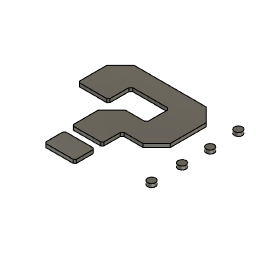
Question (Autodesk Fusion 360 design; units mm, degrees)
Autodesk Fusion 360 part; units mm, degrees
(part 1 of 2)
sketch "Schizzo1" plane through (0, 0, 0) normal (0, 0, 1) x (1, 0, 0)
  line L0 (0, 0) -> (90, 0)
  line L1 (90, 0) -> (90, 90)
  line L2 (90, 90) -> (0, 90)
  line L3 (0, 90) -> (0, 0)
  dimension "d1" = 90
  dimension "d2" = 90
  constraint horizontal L0
  constraint vertical L1
  constraint horizontal L2
  constraint vertical L3
  constraint coincident L0.start L3.end
  measures "d1" distance of L0.start L0.end
  measures "d2" distance of L0.start L2.end
ref_plane "Piano di lavoro3" through (45, 45, 11) normal (0, 0, -1) x (-1, 0, 0) in component "Cubo"
sketch "Schizzo5" plane through (0, 0, 11) normal (0, 0, 1) x (-1, 0, 0) in component "Cubo"
  arc A0 (-90, -87) -> (-87, -90) centre (-87, -87) ccw
  line L0 (-87, -90) -> (-3, -90)
  arc A1 (-3, -90) -> (0, -87) centre (-3, -87) ccw
  line L1 (0, -87) -> (0, -3)
  arc A2 (0, -3) -> (-3, 0) centre (-3, -3) ccw
  line L2 (-3, 0) -> (-87, 0)
  arc A3 (-87, 0) -> (-90, -3) centre (-87, -3) ccw
  line L3 (-90, -3) -> (-90, -87)
  line L4 (-4, -86) -> (-86, -86)
  line L5 (-86, -86) -> (-86, -4)
  line L6 (-86, -4) -> (-4, -4)
  line L7 (-4, -4) -> (-4, -86)
  dimension "d122" = 4
  dimension "d123" = 4
  dimension "d124" = 82
  dimension "d125" = 82
  constraint horizontal L4
  constraint vertical L5
  constraint horizontal L6
  constraint vertical L7
  measures "d122" distance of L2 L6
  measures "d123" distance of L1 L7
  measures "d124" distance of L4.start L6.end
  measures "d125" distance of L5.end L6.end
sketch "Schizzo6" plane through (0, 0, 11) normal (0, 0, -1) x (1, 0, 0) in component "Cubo"
  arc A0 (87, -90) -> (90, -87) centre (87, -87) ccw
  line L0 (90, -87) -> (90, -3)
  arc A1 (90, -3) -> (87, 0) centre (87, -3) ccw
  line L1 (87, 0) -> (3, 0)
  arc A2 (3, 0) -> (0, -3) centre (3, -3) ccw
  line L2 (0, -3) -> (0, -87)
  arc A3 (0, -87) -> (3, -90) centre (3, -87) ccw
  line L3 (3, -90) -> (87, -90)
  line L4 (3.5, -3.5) -> (86.5, -3.5)
  line L5 (86.5, -3.5) -> (86.5, -86.5)
  line L6 (86.5, -86.5) -> (3.5, -86.5)
  line L7 (3.5, -86.5) -> (3.5, -3.5)
  dimension "d142" = 83
  dimension "d143" = 83
  dimension "d144" = 3.5
  dimension "d145" = 3.5
  constraint horizontal L4
  constraint vertical L5
  constraint horizontal L6
  constraint vertical L7
  measures "d142" distance of L4.start L6.end
  measures "d143" distance of L4.start L4.end
  measures "d144" distance of L1 L4
  measures "d145" distance of L2 L7
sketch "Schizzo9" plane through (0, 0, 0) normal (0, -1, 0) x (1, 0, 0) in component "Cubo"
  line L0 (3, 11) -> (87, 11)
  line L1 (87, 11) -> (87, 87)
  line L2 (87, 87) -> (3, 87)
  line L3 (3, 87) -> (3, 11)
  circle A0 centre (8, 82) radius 2.5
  line L4 (87, 90) -> (3, 90)
  line L5 (0, 87) -> (0, 11)
  line L6 (45, 90) -> (45, 100)
  line L7 (0, 90) -> (0, 45)
  line L8 (0, 45) -> (-25, 45)
  circle A1 centre (82, 82) radius 2.5
  circle A2 centre (8, 8) radius 2.5
  circle A3 centre (82, 8) radius 2.5
  line L9 (24, 77.5) -> (16, 69.5)
  line L10 (16, 69.5) -> (16, 53.5)
  line L11 (16, 53.5) -> (17, 52.5)
  line L12 (17, 52.5) -> (33, 52.5)
  line L13 (33, 52.5) -> (34, 53.5)
  line L14 (34, 53.5) -> (34, 64.5)
  line L15 (34, 64.5) -> (35, 65.5)
  line L16 (35, 65.5) -> (55, 65.5)
  line L17 (55, 65.5) -> (56, 64.5)
  line L18 (56, 64.5) -> (56, 53.5)
  line L19 (56, 53.5) -> (55, 52.5)
  line L20 (55, 52.5) -> (44, 52.5)
  line L21 (44, 52.5) -> (36, 44.5)
  line L22 (36, 44.5) -> (36, 30)
  line L23 (36, 30) -> (37, 29)
  line L24 (37, 29) -> (53, 29)
  line L25 (53, 29) -> (54, 30)
  line L26 (54, 30) -> (54, 39.5)
  line L27 (54, 39.5) -> (55, 40.5)
  line L28 (55, 40.5) -> (66, 40.5)
  line L29 (66, 40.5) -> (74, 48.5)
  line L30 (74, 48.5) -> (74, 69.5)
  line L31 (74, 69.5) -> (66, 77.5)
  line L32 (66, 77.5) -> (24, 77.5)
  line L33 (36, 24) -> (37, 25)
  line L34 (37, 25) -> (53, 25)
  line L35 (53, 25) -> (54, 24)
  line L36 (54, 24) -> (54, 14)
  line L37 (54, 14) -> (53, 13)
  line L38 (53, 13) -> (37, 13)
  line L39 (37, 13) -> (36, 14)
  line L40 (36, 14) -> (36, 24)
  dimension "d49" = 5
  dimension "d50" = 8
  dimension "d51" = 8
  dimension "d52" = 45
  constraint midpoint L4 L6.start
  constraint perpendicular L4 L6
  constraint parallel L5 L7
  constraint perpendicular L5 L8
  constraint symmetric A0 L6 A1
  constraint symmetric A0 L8 A2
  constraint symmetric L8 A1 A3
  constraint perpendicular L2 L10
  constraint perpendicular L9 L11
  constraint perpendicular L10 L12
  constraint perpendicular L11 L13
  constraint perpendicular L12 L14
  constraint parallel L13 L15
  constraint perpendicular L14 L16
  constraint perpendicular L15 L17
  constraint perpendicular L16 L18
  constraint perpendicular L17 L19
  constraint perpendicular L18 L20
  constraint perpendicular L17 L21
  constraint parallel L18 L22
  constraint perpendicular L21 L23
  constraint perpendicular L22 L24
  constraint perpendicular L23 L25
  constraint perpendicular L24 L26
  constraint perpendicular L23 L27
  constraint parallel L24 L28
  constraint parallel L27 L29
  constraint vertical L30
  constraint perpendicular L29 L31
  constraint perpendicular L30 L32
  constraint parallel L9 L33
  constraint parallel L16 L34
  constraint perpendicular L33 L35
  constraint perpendicular L34 L36
  constraint perpendicular L35 L37
  constraint perpendicular L36 L38
  constraint perpendicular L37 L39
  constraint perpendicular L38 L40
  measures "d49" diameter of A0
  measures "d50" distance of A0.centre L4
  measures "d51" distance of A0.centre L5
  measures "d52" distance of L7.start L7.end
sketch "Schizzo10" plane through (45, 0, 49) normal (0, -1, 0) x (1, 0, 0) in component "Cubo"
sketch "Schizzo11" plane through (90, 0, 0) normal (1, 0, 0) x (0, 1, 0) in component "Cubo"
  line L0 (3, 11) -> (87, 11)
  line L1 (87, 11) -> (87, 87)
  line L2 (87, 87) -> (3, 87)
  line L3 (3, 87) -> (3, 11)
  line L4 (16, 69.5) -> (16, 53.5)
  line L5 (17, 52.5) -> (33, 52.5)
  line L6 (36, 24) -> (37, 25)
  line L7 (55, 52.5) -> (44, 52.5)
  line L8 (36, 44.5) -> (36, 30)
  line L9 (33, 52.5) -> (34, 53.5)
  line L10 (34, 64.5) -> (35, 65.5)
  line L11 (36, 14) -> (36, 24)
  line L12 (54, 14) -> (53, 13)
  line L13 (54, 24) -> (54, 14)
  line L14 (53, 25) -> (54, 24)
  line L15 (0, 45) -> (-25, 45)
  line L16 (36, 30) -> (37, 29)
  line L17 (56, 64.5) -> (56, 53.5)
  line L18 (24, 77.5) -> (16, 69.5)
  circle A0 centre (82, 82) radius 2.5
  line L19 (87, 90) -> (3, 90)
  line L20 (35, 65.5) -> (55, 65.5)
  line L21 (74, 48.5) -> (74, 69.5)
  line L22 (45, 90) -> (45, 100)
  line L23 (37, 25) -> (53, 25)
  line L24 (37, 29) -> (53, 29)
  line L25 (66, 40.5) -> (74, 48.5)
  line L26 (87, 87) -> (3, 87)
  line L27 (3, 11) -> (87, 11)
  line L28 (44, 52.5) -> (36, 44.5)
  line L29 (53, 13) -> (37, 13)
  line L30 (66, 77.5) -> (24, 77.5)
  circle A1 centre (82, 8) radius 2.5
  line L31 (74, 69.5) -> (66, 77.5)
  line L32 (54, 30) -> (54, 39.5)
  line L33 (53, 29) -> (54, 30)
  line L34 (54, 39.5) -> (55, 40.5)
  line L35 (37, 13) -> (36, 14)
  line L36 (56, 53.5) -> (55, 52.5)
  line L37 (55, 40.5) -> (66, 40.5)
  line L38 (55, 65.5) -> (56, 64.5)
  circle A2 centre (8, 82) radius 2.5
  line L39 (16, 53.5) -> (17, 52.5)
  line L40 (0, 90) -> (0, 45)
  circle A3 centre (8, 8) radius 2.5
  line L41 (34, 53.5) -> (34, 64.5)
  line L42 (0, 87) -> (0, 11)
  line L43 (3, 87) -> (3, 11)
  line L44 (87, 11) -> (87, 87)
  dimension "d53" = 5
  dimension "d54" = 8
  dimension "d55" = 8
  dimension "d56" = 45
  constraint midpoint L22.start L19
  constraint perpendicular L19 L22
  constraint parallel L40 L42
  constraint perpendicular L15 L42
  constraint symmetric A0 L22 A2
  constraint symmetric L15 A2 A3
  constraint symmetric L15 A0 A1
  constraint perpendicular L4 L26
  constraint perpendicular L18 L39
  constraint perpendicular L4 L5
  constraint perpendicular L9 L39
  constraint perpendicular L5 L41
  constraint parallel L9 L10
  constraint perpendicular L20 L41
  constraint perpendicular L10 L38
  constraint perpendicular L17 L20
  constraint perpendicular L36 L38
  constraint perpendicular L7 L17
  constraint perpendicular L28 L38
  constraint parallel L8 L17
  constraint perpendicular L16 L28
  constraint perpendicular L8 L24
  constraint perpendicular L16 L33
  constraint perpendicular L24 L32
  constraint perpendicular L16 L34
  constraint parallel L24 L37
  constraint parallel L25 L34
  constraint vertical L21
  constraint perpendicular L25 L31
  constraint perpendicular L21 L30
  constraint parallel L6 L18
  constraint parallel L20 L23
  constraint perpendicular L6 L14
  constraint perpendicular L13 L23
  constraint perpendicular L12 L14
  constraint perpendicular L13 L29
  constraint perpendicular L12 L35
  constraint perpendicular L11 L29
  measures "d53" diameter of A2
  measures "d54" distance of A2.centre L19
  measures "d55" distance of A2.centre L42
  measures "d56" distance of L40.start L15.start
sketch "Schizzo12" plane through (0, 0, 0) normal (-1, 0, 0) x (0, -1, 0) in component "Cubo"
  line L0 (-87, 11) -> (-3, 11)
  line L1 (-3, 11) -> (-3, 87)
  line L2 (-3, 87) -> (-87, 87)
  line L3 (-87, 87) -> (-87, 11)
  line L4 (-53, 25) -> (-37, 25)
  line L5 (-37, 13) -> (-53, 13)
  line L6 (-53, 29) -> (-37, 29)
  line L7 (-3, 90) -> (-87, 90)
  line L8 (-87, 87) -> (-87, 11)
  line L9 (-3, 11) -> (-3, 87)
  line L10 (-24, 77.5) -> (-66, 77.5)
  line L11 (-54, 24) -> (-53, 25)
  line L12 (-90, 90) -> (-90, 45)
  line L13 (-90, 45) -> (-115, 45)
  line L14 (-74, 53.5) -> (-73, 52.5)
  line L15 (-56, 64.5) -> (-55, 65.5)
  line L16 (-73, 52.5) -> (-57, 52.5)
  circle A0 centre (-82, 82) radius 2.5
  line L17 (-53, 13) -> (-54, 14)
  line L18 (-90, 87) -> (-90, 11)
  line L19 (-74, 69.5) -> (-74, 53.5)
  line L20 (-35, 52.5) -> (-46, 52.5)
  line L21 (-16, 48.5) -> (-16, 69.5)
  circle A1 centre (-82, 8) radius 2.5
  line L22 (-54, 30) -> (-53, 29)
  line L23 (-36, 39.5) -> (-35, 40.5)
  line L24 (-54, 14) -> (-54, 24)
  line L25 (-36, 30) -> (-36, 39.5)
  line L26 (-16, 69.5) -> (-24, 77.5)
  line L27 (-56, 53.5) -> (-56, 64.5)
  line L28 (-57, 52.5) -> (-56, 53.5)
  line L29 (-54, 44.5) -> (-54, 30)
  line L30 (-35, 65.5) -> (-34, 64.5)
  line L31 (-66, 77.5) -> (-74, 69.5)
  circle A2 centre (-8, 82) radius 2.5
  line L32 (-35, 40.5) -> (-24, 40.5)
  line L33 (-36, 14) -> (-37, 13)
  line L34 (-34, 53.5) -> (-35, 52.5)
  line L35 (-36, 24) -> (-36, 14)
  line L36 (-55, 65.5) -> (-35, 65.5)
  line L37 (-24, 40.5) -> (-16, 48.5)
  line L38 (-37, 29) -> (-36, 30)
  line L39 (-37, 25) -> (-36, 24)
  line L40 (-34, 64.5) -> (-34, 53.5)
  line L41 (-87, 11) -> (-3, 11)
  circle A3 centre (-8, 8) radius 2.5
  line L42 (-46, 52.5) -> (-54, 44.5)
  line L43 (-3, 87) -> (-87, 87)
  line L44 (-45, 90) -> (-45, 100)
  dimension "d57" = 5
  dimension "d58" = 8
  dimension "d59" = 8
  dimension "d60" = 45
  constraint midpoint L44.start L7
  constraint perpendicular L7 L44
  constraint parallel L12 L18
  constraint perpendicular L13 L18
  constraint symmetric A0 A2 L44
  constraint symmetric L13 A0 A1
  constraint symmetric L13 A2 A3
  constraint perpendicular L19 L43
  constraint perpendicular L14 L31
  constraint perpendicular L16 L19
  constraint perpendicular L14 L28
  constraint perpendicular L16 L27
  constraint parallel L15 L28
  constraint perpendicular L27 L36
  constraint perpendicular L15 L30
  constraint perpendicular L36 L40
  constraint perpendicular L30 L34
  constraint perpendicular L20 L40
  constraint perpendicular L30 L42
  constraint parallel L29 L40
  constraint perpendicular L22 L42
  constraint perpendicular L6 L29
  constraint perpendicular L22 L38
  constraint perpendicular L6 L25
  constraint perpendicular L22 L23
  constraint parallel L6 L32
  constraint parallel L23 L37
  constraint vertical L21
  constraint perpendicular L26 L37
  constraint perpendicular L10 L21
  constraint parallel L11 L31
  constraint parallel L4 L36
  constraint perpendicular L11 L39
  constraint perpendicular L4 L35
  constraint perpendicular L33 L39
  constraint perpendicular L5 L35
  constraint perpendicular L17 L33
  constraint perpendicular L5 L24
  measures "d57" diameter of A0
  measures "d58" distance of A0.centre L7
  measures "d59" distance of A0.centre L18
  measures "d60" distance of L12.start L12.end
sketch "Schizzo13" plane through (0, 90, 0) normal (0, 1, 0) x (-1, 0, 0) in component "Cubo"
  line L0 (-87, 11) -> (-3, 11)
  line L1 (-3, 11) -> (-3, 87)
  line L2 (-3, 87) -> (-87, 87)
  line L3 (-87, 87) -> (-87, 11)
  line L4 (-53, 25) -> (-37, 25)
  line L5 (-37, 13) -> (-53, 13)
  line L6 (-53, 29) -> (-37, 29)
  line L7 (-3, 90) -> (-87, 90)
  line L8 (-87, 87) -> (-87, 11)
  line L9 (-3, 11) -> (-3, 87)
  line L10 (-24, 77.5) -> (-66, 77.5)
  line L11 (-54, 24) -> (-53, 25)
  line L12 (-90, 90) -> (-90, 45)
  line L13 (-90, 45) -> (-115, 45)
  line L14 (-74, 53.5) -> (-73, 52.5)
  line L15 (-56, 64.5) -> (-55, 65.5)
  line L16 (-73, 52.5) -> (-57, 52.5)
  circle A0 centre (-82, 82) radius 2.5
  line L17 (-53, 13) -> (-54, 14)
  line L18 (-90, 87) -> (-90, 11)
  line L19 (-74, 69.5) -> (-74, 53.5)
  line L20 (-35, 52.5) -> (-46, 52.5)
  line L21 (-16, 48.5) -> (-16, 69.5)
  circle A1 centre (-82, 8) radius 2.5
  line L22 (-54, 30) -> (-53, 29)
  line L23 (-36, 39.5) -> (-35, 40.5)
  line L24 (-54, 14) -> (-54, 24)
  line L25 (-36, 30) -> (-36, 39.5)
  line L26 (-16, 69.5) -> (-24, 77.5)
  line L27 (-56, 53.5) -> (-56, 64.5)
  line L28 (-57, 52.5) -> (-56, 53.5)
  line L29 (-54, 44.5) -> (-54, 30)
  line L30 (-35, 65.5) -> (-34, 64.5)
  line L31 (-66, 77.5) -> (-74, 69.5)
  circle A2 centre (-8, 82) radius 2.5
  line L32 (-35, 40.5) -> (-24, 40.5)
  line L33 (-36, 14) -> (-37, 13)
  line L34 (-34, 53.5) -> (-35, 52.5)
  line L35 (-36, 24) -> (-36, 14)
  line L36 (-55, 65.5) -> (-35, 65.5)
  line L37 (-24, 40.5) -> (-16, 48.5)
  line L38 (-37, 29) -> (-36, 30)
  line L39 (-37, 25) -> (-36, 24)
  line L40 (-34, 64.5) -> (-34, 53.5)
  line L41 (-87, 11) -> (-3, 11)
  circle A3 centre (-8, 8) radius 2.5
  line L42 (-46, 52.5) -> (-54, 44.5)
  line L43 (-3, 87) -> (-87, 87)
  line L44 (-45, 90) -> (-45, 100)
  dimension "d61" = 5
  dimension "d62" = 8
  dimension "d63" = 8
  dimension "d64" = 45
  constraint midpoint L44.start L7
  constraint perpendicular L7 L44
  constraint parallel L12 L18
  constraint perpendicular L13 L18
  constraint symmetric A0 A2 L44
  constraint symmetric L13 A0 A1
  constraint symmetric L13 A2 A3
  constraint perpendicular L19 L43
  constraint perpendicular L14 L31
  constraint perpendicular L16 L19
  constraint perpendicular L14 L28
  constraint perpendicular L16 L27
  constraint parallel L15 L28
  constraint perpendicular L27 L36
  constraint perpendicular L15 L30
  constraint perpendicular L36 L40
  constraint perpendicular L30 L34
  constraint perpendicular L20 L40
  constraint perpendicular L30 L42
  constraint parallel L29 L40
  constraint perpendicular L22 L42
  constraint perpendicular L6 L29
  constraint perpendicular L22 L38
  constraint perpendicular L6 L25
  constraint perpendicular L22 L23
  constraint parallel L6 L32
  constraint parallel L23 L37
  constraint vertical L21
  constraint perpendicular L26 L37
  constraint perpendicular L10 L21
  constraint parallel L11 L31
  constraint parallel L4 L36
  constraint perpendicular L11 L39
  constraint perpendicular L4 L35
  constraint perpendicular L33 L39
  constraint perpendicular L5 L35
  constraint perpendicular L17 L33
  constraint perpendicular L5 L24
  measures "d61" diameter of A0
  measures "d62" distance of A0.centre L7
  measures "d63" distance of A0.centre L18
  measures "d64" distance of L12.start L12.end
sketch "Schizzo14" plane through (0, 0, 16) normal (0, 0, 1) x (-1, 0, 0) in component "Cubo"
  line L0 (-4, -4) -> (-86, -4)
  line L1 (-86, -4) -> (-86, -86)
  line L2 (-4, -86) -> (-4, -4)
  line L3 (0, -90) -> (0, -45)
  line L4 (0, -45) -> (11, -45)
  arc A0 (-32.6706, -81.0285) -> (-30.0706, -81.0285) centre (-31.3706, -82.2) ccw
  arc A1 (-35.024, -79.1) -> (-35.024, -80.3) centre (-36.1206, -79.7) ccw
  arc A2 (-27.7171, -80.3) -> (-27.7171, -79.1) centre (-26.6206, -79.7) ccw
  line L5 (-28.8206, -77.5) -> (-30.0706, -77.5)
  line L6 (-32.6706, -77.5) -> (-33.9206, -77.5)
  line L7 (-27.7171, -71.95) -> (-28.8206, -71.95)
  line L8 (-33.9206, -71.95) -> (-35.024, -71.95)
  line L9 (-35.024, -70.75) -> (-33.9206, -70.75)
  line L10 (-28.8206, -70.75) -> (-27.7171, -70.75)
  arc A3 (-27.7171, -71.95) -> (-27.7171, -70.75) centre (-26.6206, -71.35) ccw
  arc A4 (-35.024, -70.75) -> (-35.024, -71.95) centre (-36.1206, -71.35) ccw
  line L11 (-33.9206, -77.5) -> (-33.9206, -71.95)
  line L12 (-33.9206, -70.75) -> (-33.9206, -65.2)
  line L13 (-33.9206, -65.2) -> (-32.6706, -65.2)
  line L14 (-30.0706, -65.2) -> (-28.8206, -65.2)
  line L15 (-35.024, -63.6) -> (-32.6706, -63.6)
  line L16 (-30.0706, -63.6) -> (-27.7171, -63.6)
  arc A5 (-35.024, -62.4) -> (-35.024, -63.6) centre (-36.1206, -63) ccw
  arc A6 (-30.0706, -61.6715) -> (-32.6706, -61.6715) centre (-31.3706, -60.5) ccw
  line L17 (-27.7171, -62.4) -> (-30.0706, -62.4)
  line L18 (-32.6706, -62.4) -> (-35.024, -62.4)
  line L19 (-32.6706, -65.2) -> (-32.6706, -63.6)
  line L20 (-32.6706, -62.4) -> (-32.6706, -61.6715)
  line L21 (-30.0706, -61.6715) -> (-30.0706, -62.4)
  line L22 (-30.0706, -63.6) -> (-30.0706, -65.2)
  arc A7 (-27.7171, -63.6) -> (-27.7171, -62.4) centre (-26.6206, -63) ccw
  line L23 (-28.8206, -65.2) -> (-28.8206, -70.75)
  line L24 (-28.8206, -71.95) -> (-28.8206, -77.5)
  line L25 (-30.0706, -81.0285) -> (-30.0706, -80.3)
  line L26 (-30.0706, -79.1) -> (-30.0706, -77.5)
  line L27 (-27.7171, -80.3) -> (-30.0706, -80.3)
  line L28 (-32.6706, -80.3) -> (-35.024, -80.3)
  line L29 (-35.024, -79.1) -> (-32.6706, -79.1)
  line L30 (-30.0706, -79.1) -> (-27.7171, -79.1)
  line L31 (-32.6706, -77.5) -> (-32.6706, -79.1)
  line L32 (-32.6706, -80.3) -> (-32.6706, -81.0285)
  line L33 (-43.6956, -79.1) -> (-43.6956, -77.5)
  line L34 (-46.2956, -77.5) -> (-46.2956, -79.1)
  line L35 (-41.3421, -80.3) -> (-43.6956, -80.3)
  line L36 (-46.2956, -80.3) -> (-48.649, -80.3)
  line L37 (-42.4456, -77.5) -> (-43.6956, -77.5)
  line L38 (-46.2956, -77.5) -> (-47.5456, -77.5)
  line L39 (-48.649, -79.1) -> (-46.2956, -79.1)
  line L40 (-43.6956, -79.1) -> (-41.3421, -79.1)
  arc A8 (-41.3421, -80.3) -> (-41.3421, -79.1) centre (-40.2456, -79.7) ccw
  arc A9 (-48.649, -79.1) -> (-48.649, -80.3) centre (-49.7456, -79.7) ccw
  line L41 (-47.5456, -77.5) -> (-47.5456, -71.95)
  line L42 (-47.5456, -70.75) -> (-47.5456, -65.2)
  line L43 (-41.3421, -71.95) -> (-42.4456, -71.95)
  line L44 (-47.5456, -71.95) -> (-48.649, -71.95)
  line L45 (-48.649, -70.75) -> (-47.5456, -70.75)
  line L46 (-42.4456, -70.75) -> (-41.3421, -70.75)
  arc A10 (-48.649, -70.75) -> (-48.649, -71.95) centre (-49.7456, -71.35) ccw
  arc A11 (-41.3421, -71.95) -> (-41.3421, -70.75) centre (-40.2456, -71.35) ccw
  line L47 (-47.5456, -65.2) -> (-46.2956, -65.2)
  line L48 (-43.6956, -65.2) -> (-42.4456, -65.2)
  line L49 (-41.3421, -62.4) -> (-43.6956, -62.4)
  line L50 (-46.2956, -62.4) -> (-48.649, -62.4)
  arc A12 (-43.6956, -61.6715) -> (-46.2956, -61.6715) centre (-44.9956, -60.5) ccw
  line L51 (-48.649, -63.6) -> (-46.2956, -63.6)
  line L52 (-43.6956, -63.6) -> (-41.3421, -63.6)
  line L53 (-43.6956, -61.6715) -> (-43.6956, -62.4)
  line L54 (-43.6956, -63.6) -> (-43.6956, -65.2)
  arc A13 (-41.3421, -63.6) -> (-41.3421, -62.4) centre (-40.2456, -63) ccw
  line L55 (-46.2956, -65.2) -> (-46.2956, -63.6)
  line L56 (-46.2956, -62.4) -> (-46.2956, -61.6715)
  arc A14 (-48.649, -62.4) -> (-48.649, -63.6) centre (-49.7456, -63) ccw
  arc A15 (-54.9671, -63.6) -> (-54.9671, -62.4) centre (-53.8706, -63) ccw
  line L57 (-54.9671, -62.4) -> (-57.3206, -62.4)
  line L58 (-59.9206, -62.4) -> (-62.274, -62.4)
  arc A16 (-57.3206, -61.6715) -> (-59.9206, -61.6715) centre (-58.6206, -60.5) ccw
  line L59 (-59.9206, -65.2) -> (-59.9206, -63.6)
  line L60 (-59.9206, -62.4) -> (-59.9206, -61.6715)
  line L61 (-62.274, -63.6) -> (-59.9206, -63.6)
  line L62 (-57.3206, -63.6) -> (-54.9671, -63.6)
  line L63 (-61.1706, -65.2) -> (-59.9206, -65.2)
  line L64 (-57.3206, -65.2) -> (-56.0706, -65.2)
  arc A17 (-62.274, -62.4) -> (-62.274, -63.6) centre (-63.3706, -63) ccw
  line L65 (-61.1706, -77.5) -> (-61.1706, -71.95)
  line L66 (-61.1706, -70.75) -> (-61.1706, -65.2)
  line L67 (-54.9671, -71.95) -> (-56.0706, -71.95)
  line L68 (-61.1706, -71.95) -> (-62.274, -71.95)
  line L69 (-62.274, -70.75) -> (-61.1706, -70.75)
  line L70 (-56.0706, -70.75) -> (-54.9671, -70.75)
  arc A18 (-62.274, -70.75) -> (-62.274, -71.95) centre (-63.3706, -71.35) ccw
  line L71 (-56.0706, -65.2) -> (-56.0706, -70.75)
  line L72 (-56.0706, -71.95) -> (-56.0706, -77.5)
  arc A19 (-54.9671, -71.95) -> (-54.9671, -70.75) centre (-53.8706, -71.35) ccw
  line L73 (-56.0706, -77.5) -> (-57.3206, -77.5)
  line L74 (-59.9206, -77.5) -> (-61.1706, -77.5)
  line L75 (-62.274, -79.1) -> (-59.9206, -79.1)
  line L76 (-57.3206, -79.1) -> (-54.9671, -79.1)
  arc A20 (-59.9206, -81.0285) -> (-57.3206, -81.0285) centre (-58.6206, -82.2) ccw
  line L77 (-54.9671, -80.3) -> (-57.3206, -80.3)
  line L78 (-59.9206, -80.3) -> (-62.274, -80.3)
  arc A21 (-54.9671, -80.3) -> (-54.9671, -79.1) centre (-53.8706, -79.7) ccw
  arc A22 (-62.274, -79.1) -> (-62.274, -80.3) centre (-63.3706, -79.7) ccw
  line L79 (-59.9206, -77.5) -> (-59.9206, -79.1)
  line L80 (-59.9206, -80.3) -> (-59.9206, -81.0285)
  line L81 (-57.3206, -81.0285) -> (-57.3206, -80.3)
  line L82 (-57.3206, -79.1) -> (-57.3206, -77.5)
  arc A23 (-73.5456, -81.0285) -> (-70.9456, -81.0285) centre (-72.2456, -82.2) ccw
  line L83 (-68.5921, -80.3) -> (-70.9456, -80.3)
  line L84 (-73.5456, -80.3) -> (-75.899, -80.3)
  arc A24 (-68.5921, -80.3) -> (-68.5921, -79.1) centre (-67.4956, -79.7) ccw
  line L85 (-75.899, -79.1) -> (-73.5456, -79.1)
  line L86 (-70.9456, -79.1) -> (-68.5921, -79.1)
  line L87 (-69.6956, -77.5) -> (-70.9456, -77.5)
  line L88 (-73.5456, -77.5) -> (-74.7956, -77.5)
  line L89 (-73.5456, -77.5) -> (-73.5456, -79.1)
  line L90 (-73.5456, -80.3) -> (-73.5456, -81.0285)
  arc A25 (-75.899, -79.1) -> (-75.899, -80.3) centre (-76.9956, -79.7) ccw
  line L91 (-68.5921, -71.95) -> (-69.6956, -71.95)
  line L92 (-74.7956, -71.95) -> (-75.899, -71.95)
  arc A26 (-75.899, -70.75) -> (-75.899, -71.95) centre (-76.9956, -71.35) ccw
  line L93 (-74.7956, -77.5) -> (-74.7956, -71.95)
  line L94 (-74.7956, -70.75) -> (-74.7956, -65.2)
  line L95 (-69.6956, -65.2) -> (-69.6956, -70.75)
  line L96 (-69.6956, -71.95) -> (-69.6956, -77.5)
  arc A27 (-68.5921, -71.95) -> (-68.5921, -70.75) centre (-67.4956, -71.35) ccw
  line L97 (-74.7956, -65.2) -> (-73.5456, -65.2)
  line L98 (-70.9456, -65.2) -> (-69.6956, -65.2)
  line L99 (-75.899, -70.75) -> (-74.7956, -70.75)
  line L100 (-69.6956, -70.75) -> (-68.5921, -70.75)
  line L101 (-75.899, -63.6) -> (-73.5456, -63.6)
  line L102 (-70.9456, -63.6) -> (-68.5921, -63.6)
  line L103 (-73.5456, -65.2) -> (-73.5456, -63.6)
  line L104 (-73.5456, -62.4) -> (-73.5456, -61.6715)
  line L105 (-68.5921, -62.4) -> (-70.9456, -62.4)
  line L106 (-73.5456, -62.4) -> (-75.899, -62.4)
  arc A28 (-70.9456, -61.6715) -> (-73.5456, -61.6715) centre (-72.2456, -60.5) ccw
  arc A29 (-68.5921, -63.6) -> (-68.5921, -62.4) centre (-67.4956, -63) ccw
  line L107 (-70.9456, -61.6715) -> (-70.9456, -62.4)
  line L108 (-70.9456, -63.6) -> (-70.9456, -65.2)
  arc A30 (-75.899, -62.4) -> (-75.899, -63.6) centre (-76.9956, -63) ccw
  line L109 (-70.9456, -81.0285) -> (-70.9456, -80.3)
  line L110 (-70.9456, -79.1) -> (-70.9456, -77.5)
  line L111 (-57.3206, -61.6715) -> (-57.3206, -62.4)
  line L112 (-57.3206, -63.6) -> (-57.3206, -65.2)
  line L113 (-42.4456, -65.2) -> (-42.4456, -70.75)
  line L114 (-42.4456, -71.95) -> (-42.4456, -77.5)
  line L115 (-43.6956, -80.3) -> (-43.6956, -81.0285)
  line L116 (-46.2956, -80.3) -> (-46.2956, -81.0285)
  arc A31 (-46.2956, -81.0285) -> (-43.6956, -81.0285) centre (-44.9956, -82.2) ccw
  line L117 (-27.7171, -36.05) -> (-30.0706, -36.05)
  line L118 (-59.9206, -38.85) -> (-59.9206, -37.25)
  line L119 (-68.5921, -36.05) -> (-70.9456, -36.05)
  line L120 (-43.6956, -35.3215) -> (-43.6956, -36.05)
  arc A32 (-75.899, -52.75) -> (-75.899, -53.95) centre (-76.9956, -53.35) ccw
  line L121 (-30.0706, -38.85) -> (-28.8206, -38.85)
  line L122 (-75.899, -52.75) -> (-73.5456, -52.75)
  arc A33 (-68.5921, -37.25) -> (-68.5921, -36.05) centre (-67.4956, -36.65) ccw
  arc A34 (-48.649, -36.05) -> (-48.649, -37.25) centre (-49.7456, -36.65) ccw
  line L123 (-59.9206, -36.05) -> (-62.274, -36.05)
  line L124 (-46.2956, -36.05) -> (-48.649, -36.05)
  line L125 (-54.9671, -36.05) -> (-57.3206, -36.05)
  arc A35 (-46.2956, -54.6785) -> (-43.6956, -54.6785) centre (-44.9956, -55.85) ccw
  line L126 (-57.3206, -37.25) -> (-57.3206, -38.85)
  arc A36 (-54.9671, -37.25) -> (-54.9671, -36.05) centre (-53.8706, -36.65) ccw
  line L127 (-68.5921, -53.95) -> (-70.9456, -53.95)
  line L128 (-32.6706, -36.05) -> (-35.024, -36.05)
  line L129 (-30.0706, -35.3215) -> (-30.0706, -36.05)
  arc A37 (-57.3206, -35.3215) -> (-59.9206, -35.3215) centre (-58.6206, -34.15) ccw
  arc A38 (-30.0706, -35.3215) -> (-32.6706, -35.3215) centre (-31.3706, -34.15) ccw
  line L130 (-32.6706, -38.85) -> (-32.6706, -37.25)
  line L131 (-46.2956, -38.85) -> (-46.2956, -37.25)
  line L132 (-47.5456, -38.85) -> (-46.2956, -38.85)
  line L133 (-59.9206, -36.05) -> (-59.9206, -35.3215)
  line L134 (-57.3206, -37.25) -> (-54.9671, -37.25)
  line L135 (-73.5456, -53.95) -> (-75.899, -53.95)
  line L136 (-69.6956, -51.15) -> (-70.9456, -51.15)
  line L137 (-30.0706, -37.25) -> (-30.0706, -38.85)
  arc A39 (-62.274, -36.05) -> (-62.274, -37.25) centre (-63.3706, -36.65) ccw
  line L138 (-73.5456, -36.05) -> (-75.899, -36.05)
  arc A40 (-41.3421, -37.25) -> (-41.3421, -36.05) centre (-40.2456, -36.65) ccw
  line L139 (-35.024, -37.25) -> (-32.6706, -37.25)
  line L140 (-48.649, -37.25) -> (-46.2956, -37.25)
  line L141 (-62.274, -37.25) -> (-59.9206, -37.25)
  arc A41 (-43.6956, -35.3215) -> (-46.2956, -35.3215) centre (-44.9956, -34.15) ccw
  line L142 (-57.3206, -35.3215) -> (-57.3206, -36.05)
  line L143 (-61.1706, -38.85) -> (-59.9206, -38.85)
  line L144 (-57.3206, -38.85) -> (-56.0706, -38.85)
  line L145 (-46.2956, -36.05) -> (-46.2956, -35.3215)
  line L146 (-75.899, -44.4) -> (-74.7956, -44.4)
  line L147 (-59.9206, -51.15) -> (-59.9206, -52.75)
  line L148 (-46.2956, -51.15) -> (-47.5456, -51.15)
  line L149 (-73.5456, -51.15) -> (-73.5456, -52.75)
  arc A42 (-48.649, -52.75) -> (-48.649, -53.95) centre (-49.7456, -53.35) ccw
  line L150 (-35.024, -44.4) -> (-33.9206, -44.4)
  line L151 (-48.649, -52.75) -> (-46.2956, -52.75)
  arc A43 (-32.6706, -54.6785) -> (-30.0706, -54.6785) centre (-31.3706, -55.85) ccw
  line L152 (-73.5456, -51.15) -> (-74.7956, -51.15)
  line L153 (-47.5456, -51.15) -> (-47.5456, -45.6)
  arc A44 (-35.024, -44.4) -> (-35.024, -45.6) centre (-36.1206, -45) ccw
  line L154 (-62.274, -52.75) -> (-59.9206, -52.75)
  arc A45 (-54.9671, -53.95) -> (-54.9671, -52.75) centre (-53.8706, -53.35) ccw
  line L155 (-33.9206, -44.4) -> (-33.9206, -38.85)
  line L156 (-46.2956, -51.15) -> (-46.2956, -52.75)
  line L157 (-28.8206, -38.85) -> (-28.8206, -44.4)
  line L158 (-70.9456, -54.6785) -> (-70.9456, -53.95)
  arc A46 (-75.899, -36.05) -> (-75.899, -37.25) centre (-76.9956, -36.65) ccw
  line L159 (-70.9456, -35.3215) -> (-70.9456, -36.05)
  line L160 (-57.3206, -54.6785) -> (-57.3206, -53.95)
  line L161 (-73.5456, -53.95) -> (-73.5456, -54.6785)
  arc A47 (-41.3421, -45.6) -> (-41.3421, -44.4) centre (-40.2456, -45) ccw
  line L162 (-27.7171, -45.6) -> (-28.8206, -45.6)
  line L163 (-42.4456, -44.4) -> (-41.3421, -44.4)
  line L164 (-28.8206, -51.15) -> (-30.0706, -51.15)
  arc A48 (-62.274, -44.4) -> (-62.274, -45.6) centre (-63.3706, -45) ccw
  arc A49 (-59.9206, -54.6785) -> (-57.3206, -54.6785) centre (-58.6206, -55.85) ccw
  line L165 (-73.5456, -38.85) -> (-73.5456, -37.25)
  line L166 (-70.9456, -38.85) -> (-69.6956, -38.85)
  line L167 (-68.5921, -45.6) -> (-69.6956, -45.6)
  line L168 (-42.4456, -51.15) -> (-43.6956, -51.15)
  line L169 (-56.0706, -45.6) -> (-56.0706, -51.15)
  line L170 (-32.6706, -51.15) -> (-32.6706, -52.75)
  line L171 (-61.1706, -45.6) -> (-62.274, -45.6)
  arc A50 (-73.5456, -54.6785) -> (-70.9456, -54.6785) centre (-72.2456, -55.85) ccw
  line L172 (-43.6956, -52.75) -> (-41.3421, -52.75)
  line L173 (-70.9456, -37.25) -> (-70.9456, -38.85)
  arc A51 (-27.7171, -45.6) -> (-27.7171, -44.4) centre (-26.6206, -45) ccw
  line L174 (-69.6956, -45.6) -> (-69.6956, -51.15)
  line L175 (-28.8206, -45.6) -> (-28.8206, -51.15)
  line L176 (-46.2956, -53.95) -> (-46.2956, -54.6785)
  line L177 (-70.9456, -52.75) -> (-70.9456, -51.15)
  line L178 (-41.3421, -45.6) -> (-42.4456, -45.6)
  line L179 (-32.6706, -53.95) -> (-35.024, -53.95)
  line L180 (-62.274, -44.4) -> (-61.1706, -44.4)
  line L181 (-35.024, -52.75) -> (-32.6706, -52.75)
  line L182 (-30.0706, -52.75) -> (-30.0706, -51.15)
  line L183 (-56.0706, -44.4) -> (-54.9671, -44.4)
  line L184 (-41.3421, -53.95) -> (-43.6956, -53.95)
  line L185 (-30.0706, -54.6785) -> (-30.0706, -53.95)
  line L186 (-59.9206, -51.15) -> (-61.1706, -51.15)
  line L187 (-43.6956, -53.95) -> (-43.6956, -54.6785)
  line L188 (-54.9671, -53.95) -> (-57.3206, -53.95)
  line L189 (-32.6706, -51.15) -> (-33.9206, -51.15)
  arc A52 (-27.7171, -53.95) -> (-27.7171, -52.75) centre (-26.6206, -53.35) ccw
  line L190 (-33.9206, -45.6) -> (-35.024, -45.6)
  line L191 (-32.6706, -53.95) -> (-32.6706, -54.6785)
  line L192 (-57.3206, -52.75) -> (-54.9671, -52.75)
  arc A53 (-62.274, -52.75) -> (-62.274, -53.95) centre (-63.3706, -53.35) ccw
  arc A54 (-54.9671, -45.6) -> (-54.9671, -44.4) centre (-53.8706, -45) ccw
  arc A55 (-41.3421, -53.95) -> (-41.3421, -52.75) centre (-40.2456, -53.35) ccw
  line L193 (-43.6956, -52.75) -> (-43.6956, -51.15)
  line L194 (-27.7171, -53.95) -> (-30.0706, -53.95)
  line L195 (-28.8206, -44.4) -> (-27.7171, -44.4)
  arc A56 (-35.024, -52.75) -> (-35.024, -53.95) centre (-36.1206, -53.35) ccw
  line L196 (-30.0706, -52.75) -> (-27.7171, -52.75)
  line L197 (-42.4456, -45.6) -> (-42.4456, -51.15)
  arc A57 (-48.649, -44.4) -> (-48.649, -45.6) centre (-49.7456, -45) ccw
  line L198 (-33.9206, -51.15) -> (-33.9206, -45.6)
  arc A58 (-35.024, -36.05) -> (-35.024, -37.25) centre (-36.1206, -36.65) ccw
  line L199 (-74.7956, -38.85) -> (-73.5456, -38.85)
  line L200 (-56.0706, -51.15) -> (-57.3206, -51.15)
  line L201 (-57.3206, -52.75) -> (-57.3206, -51.15)
  line L202 (-30.0706, -37.25) -> (-27.7171, -37.25)
  arc A59 (-75.899, -44.4) -> (-75.899, -45.6) centre (-76.9956, -45) ccw
  line L203 (-74.7956, -51.15) -> (-74.7956, -45.6)
  arc A60 (-68.5921, -45.6) -> (-68.5921, -44.4) centre (-67.4956, -45) ccw
  line L204 (-74.7956, -45.6) -> (-75.899, -45.6)
  line L205 (-70.9456, -52.75) -> (-68.5921, -52.75)
  line L206 (-56.0706, -38.85) -> (-56.0706, -44.4)
  line L207 (-42.4456, -38.85) -> (-42.4456, -44.4)
  line L208 (-59.9206, -53.95) -> (-62.274, -53.95)
  line L209 (-46.2956, -53.95) -> (-48.649, -53.95)
  line L210 (-54.9671, -45.6) -> (-56.0706, -45.6)
  line L211 (-43.6956, -38.85) -> (-42.4456, -38.85)
  line L212 (-61.1706, -51.15) -> (-61.1706, -45.6)
  line L213 (-48.649, -44.4) -> (-47.5456, -44.4)
  line L214 (-61.1706, -44.4) -> (-61.1706, -38.85)
  line L215 (-33.9206, -38.85) -> (-32.6706, -38.85)
  line L216 (-70.9456, -37.25) -> (-68.5921, -37.25)
  arc A61 (-70.9456, -35.3215) -> (-73.5456, -35.3215) centre (-72.2456, -34.15) ccw
  line L217 (-47.5456, -45.6) -> (-48.649, -45.6)
  line L218 (-73.5456, -36.05) -> (-73.5456, -35.3215)
  line L219 (-43.6956, -37.25) -> (-43.6956, -38.85)
  arc A62 (-68.5921, -53.95) -> (-68.5921, -52.75) centre (-67.4956, -53.35) ccw
  line L220 (-69.6956, -44.4) -> (-68.5921, -44.4)
  line L221 (-32.6706, -36.05) -> (-32.6706, -35.3215)
  line L222 (-74.7956, -44.4) -> (-74.7956, -38.85)
  line L223 (-75.899, -37.25) -> (-73.5456, -37.25)
  line L224 (-43.6956, -37.25) -> (-41.3421, -37.25)
  line L225 (-41.3421, -36.05) -> (-43.6956, -36.05)
  arc A63 (-27.7171, -37.25) -> (-27.7171, -36.05) centre (-26.6206, -36.65) ccw
  line L226 (-69.6956, -38.85) -> (-69.6956, -44.4)
  line L227 (-47.5456, -44.4) -> (-47.5456, -38.85)
  line L228 (-59.9206, -53.95) -> (-59.9206, -54.6785)
  line L229 (-27.7171, -9.7) -> (-30.0706, -9.7)
  line L230 (-59.9206, -12.5) -> (-59.9206, -10.9)
  line L231 (-68.5921, -9.7) -> (-70.9456, -9.7)
  line L232 (-43.6956, -8.9715) -> (-43.6956, -9.7)
  arc A64 (-75.899, -26.4) -> (-75.899, -27.6) centre (-76.9956, -27) ccw
  line L233 (-30.0706, -12.5) -> (-28.8206, -12.5)
  line L234 (-75.899, -26.4) -> (-73.5456, -26.4)
  arc A65 (-68.5921, -10.9) -> (-68.5921, -9.7) centre (-67.4956, -10.3) ccw
  arc A66 (-48.649, -9.7) -> (-48.649, -10.9) centre (-49.7456, -10.3) ccw
  line L235 (-59.9206, -9.7) -> (-62.274, -9.7)
  line L236 (-46.2956, -9.7) -> (-48.649, -9.7)
  line L237 (-54.9671, -9.7) -> (-57.3206, -9.7)
  arc A67 (-46.2956, -28.3285) -> (-43.6956, -28.3285) centre (-44.9956, -29.5) ccw
  line L238 (-57.3206, -10.9) -> (-57.3206, -12.5)
  arc A68 (-54.9671, -10.9) -> (-54.9671, -9.7) centre (-53.8706, -10.3) ccw
  line L239 (-68.5921, -27.6) -> (-70.9456, -27.6)
  line L240 (-32.6706, -9.7) -> (-35.024, -9.7)
  line L241 (-30.0706, -8.9715) -> (-30.0706, -9.7)
  arc A69 (-57.3206, -8.9715) -> (-59.9206, -8.9715) centre (-58.6206, -7.8) ccw
  arc A70 (-30.0706, -8.9715) -> (-32.6706, -8.9715) centre (-31.3706, -7.8) ccw
  line L242 (-32.6706, -12.5) -> (-32.6706, -10.9)
  line L243 (-46.2956, -12.5) -> (-46.2956, -10.9)
  line L244 (-47.5456, -12.5) -> (-46.2956, -12.5)
  line L245 (-59.9206, -9.7) -> (-59.9206, -8.9715)
  line L246 (-57.3206, -10.9) -> (-54.9671, -10.9)
  line L247 (-73.5456, -27.6) -> (-75.899, -27.6)
  line L248 (-69.6956, -24.8) -> (-70.9456, -24.8)
  line L249 (-30.0706, -10.9) -> (-30.0706, -12.5)
  arc A71 (-62.274, -9.7) -> (-62.274, -10.9) centre (-63.3706, -10.3) ccw
  line L250 (-73.5456, -9.7) -> (-75.899, -9.7)
  arc A72 (-41.3421, -10.9) -> (-41.3421, -9.7) centre (-40.2456, -10.3) ccw
  line L251 (-35.024, -10.9) -> (-32.6706, -10.9)
  line L252 (-48.649, -10.9) -> (-46.2956, -10.9)
  line L253 (-62.274, -10.9) -> (-59.9206, -10.9)
  arc A73 (-43.6956, -8.9715) -> (-46.2956, -8.9715) centre (-44.9956, -7.8) ccw
  line L254 (-57.3206, -8.9715) -> (-57.3206, -9.7)
  line L255 (-61.1706, -12.5) -> (-59.9206, -12.5)
  line L256 (-57.3206, -12.5) -> (-56.0706, -12.5)
  line L257 (-46.2956, -9.7) -> (-46.2956, -8.9715)
  line L258 (-75.899, -18.05) -> (-74.7956, -18.05)
  line L259 (-59.9206, -24.8) -> (-59.9206, -26.4)
  line L260 (-46.2956, -24.8) -> (-47.5456, -24.8)
  line L261 (-73.5456, -24.8) -> (-73.5456, -26.4)
  arc A74 (-48.649, -26.4) -> (-48.649, -27.6) centre (-49.7456, -27) ccw
  line L262 (-35.024, -18.05) -> (-33.9206, -18.05)
  line L263 (-48.649, -26.4) -> (-46.2956, -26.4)
  arc A75 (-32.6706, -28.3285) -> (-30.0706, -28.3285) centre (-31.3706, -29.5) ccw
  line L264 (-73.5456, -24.8) -> (-74.7956, -24.8)
  line L265 (-47.5456, -24.8) -> (-47.5456, -19.25)
  arc A76 (-35.024, -18.05) -> (-35.024, -19.25) centre (-36.1206, -18.65) ccw
  line L266 (-62.274, -26.4) -> (-59.9206, -26.4)
  arc A77 (-54.9671, -27.6) -> (-54.9671, -26.4) centre (-53.8706, -27) ccw
  line L267 (-33.9206, -18.05) -> (-33.9206, -12.5)
  line L268 (-46.2956, -24.8) -> (-46.2956, -26.4)
  line L269 (-28.8206, -12.5) -> (-28.8206, -18.05)
  line L270 (-70.9456, -28.3285) -> (-70.9456, -27.6)
  arc A78 (-75.899, -9.7) -> (-75.899, -10.9) centre (-76.9956, -10.3) ccw
  line L271 (-70.9456, -8.9715) -> (-70.9456, -9.7)
  line L272 (-57.3206, -28.3285) -> (-57.3206, -27.6)
  line L273 (-73.5456, -27.6) -> (-73.5456, -28.3285)
  arc A79 (-41.3421, -19.25) -> (-41.3421, -18.05) centre (-40.2456, -18.65) ccw
  line L274 (-27.7171, -19.25) -> (-28.8206, -19.25)
  line L275 (-42.4456, -18.05) -> (-41.3421, -18.05)
  line L276 (-28.8206, -24.8) -> (-30.0706, -24.8)
  arc A80 (-62.274, -18.05) -> (-62.274, -19.25) centre (-63.3706, -18.65) ccw
  arc A81 (-59.9206, -28.3285) -> (-57.3206, -28.3285) centre (-58.6206, -29.5) ccw
  line L277 (-73.5456, -12.5) -> (-73.5456, -10.9)
  line L278 (-70.9456, -12.5) -> (-69.6956, -12.5)
  line L279 (-68.5921, -19.25) -> (-69.6956, -19.25)
  line L280 (-42.4456, -24.8) -> (-43.6956, -24.8)
  line L281 (-56.0706, -19.25) -> (-56.0706, -24.8)
  line L282 (-32.6706, -24.8) -> (-32.6706, -26.4)
  line L283 (-61.1706, -19.25) -> (-62.274, -19.25)
  arc A82 (-73.5456, -28.3285) -> (-70.9456, -28.3285) centre (-72.2456, -29.5) ccw
  line L284 (-43.6956, -26.4) -> (-41.3421, -26.4)
  line L285 (-70.9456, -10.9) -> (-70.9456, -12.5)
  arc A83 (-27.7171, -19.25) -> (-27.7171, -18.05) centre (-26.6206, -18.65) ccw
  line L286 (-69.6956, -19.25) -> (-69.6956, -24.8)
  line L287 (-28.8206, -19.25) -> (-28.8206, -24.8)
  line L288 (-46.2956, -27.6) -> (-46.2956, -28.3285)
  line L289 (-70.9456, -26.4) -> (-70.9456, -24.8)
  line L290 (-41.3421, -19.25) -> (-42.4456, -19.25)
  line L291 (-32.6706, -27.6) -> (-35.024, -27.6)
  line L292 (-62.274, -18.05) -> (-61.1706, -18.05)
  line L293 (-35.024, -26.4) -> (-32.6706, -26.4)
  line L294 (-30.0706, -26.4) -> (-30.0706, -24.8)
  line L295 (-56.0706, -18.05) -> (-54.9671, -18.05)
  line L296 (-41.3421, -27.6) -> (-43.6956, -27.6)
  line L297 (-30.0706, -28.3285) -> (-30.0706, -27.6)
  line L298 (-59.9206, -24.8) -> (-61.1706, -24.8)
  line L299 (-43.6956, -27.6) -> (-43.6956, -28.3285)
  line L300 (-54.9671, -27.6) -> (-57.3206, -27.6)
  line L301 (-32.6706, -24.8) -> (-33.9206, -24.8)
  arc A84 (-27.7171, -27.6) -> (-27.7171, -26.4) centre (-26.6206, -27) ccw
  line L302 (-33.9206, -19.25) -> (-35.024, -19.25)
  line L303 (-32.6706, -27.6) -> (-32.6706, -28.3285)
  line L304 (-57.3206, -26.4) -> (-54.9671, -26.4)
  arc A85 (-62.274, -26.4) -> (-62.274, -27.6) centre (-63.3706, -27) ccw
  arc A86 (-54.9671, -19.25) -> (-54.9671, -18.05) centre (-53.8706, -18.65) ccw
  arc A87 (-41.3421, -27.6) -> (-41.3421, -26.4) centre (-40.2456, -27) ccw
  line L305 (-43.6956, -26.4) -> (-43.6956, -24.8)
  line L306 (-27.7171, -27.6) -> (-30.0706, -27.6)
  line L307 (-28.8206, -18.05) -> (-27.7171, -18.05)
  arc A88 (-35.024, -26.4) -> (-35.024, -27.6) centre (-36.1206, -27) ccw
  line L308 (-30.0706, -26.4) -> (-27.7171, -26.4)
  line L309 (-42.4456, -19.25) -> (-42.4456, -24.8)
  arc A89 (-48.649, -18.05) -> (-48.649, -19.25) centre (-49.7456, -18.65) ccw
  line L310 (-33.9206, -24.8) -> (-33.9206, -19.25)
  arc A90 (-35.024, -9.7) -> (-35.024, -10.9) centre (-36.1206, -10.3) ccw
  line L311 (-74.7956, -12.5) -> (-73.5456, -12.5)
  line L312 (-56.0706, -24.8) -> (-57.3206, -24.8)
  line L313 (-57.3206, -26.4) -> (-57.3206, -24.8)
  line L314 (-30.0706, -10.9) -> (-27.7171, -10.9)
  arc A91 (-75.899, -18.05) -> (-75.899, -19.25) centre (-76.9956, -18.65) ccw
  line L315 (-74.7956, -24.8) -> (-74.7956, -19.25)
  arc A92 (-68.5921, -19.25) -> (-68.5921, -18.05) centre (-67.4956, -18.65) ccw
  line L316 (-74.7956, -19.25) -> (-75.899, -19.25)
  line L317 (-70.9456, -26.4) -> (-68.5921, -26.4)
  line L318 (-56.0706, -12.5) -> (-56.0706, -18.05)
  line L319 (-42.4456, -12.5) -> (-42.4456, -18.05)
  line L320 (-59.9206, -27.6) -> (-62.274, -27.6)
  line L321 (-46.2956, -27.6) -> (-48.649, -27.6)
  line L322 (-54.9671, -19.25) -> (-56.0706, -19.25)
  line L323 (-43.6956, -12.5) -> (-42.4456, -12.5)
  line L324 (-61.1706, -24.8) -> (-61.1706, -19.25)
  line L325 (-48.649, -18.05) -> (-47.5456, -18.05)
  line L326 (-61.1706, -18.05) -> (-61.1706, -12.5)
  line L327 (-33.9206, -12.5) -> (-32.6706, -12.5)
  line L328 (-70.9456, -10.9) -> (-68.5921, -10.9)
  arc A93 (-70.9456, -8.9715) -> (-73.5456, -8.9715) centre (-72.2456, -7.8) ccw
  line L329 (-47.5456, -19.25) -> (-48.649, -19.25)
  line L330 (-73.5456, -9.7) -> (-73.5456, -8.9715)
  line L331 (-43.6956, -10.9) -> (-43.6956, -12.5)
  arc A94 (-68.5921, -27.6) -> (-68.5921, -26.4) centre (-67.4956, -27) ccw
  line L332 (-69.6956, -18.05) -> (-68.5921, -18.05)
  line L333 (-32.6706, -9.7) -> (-32.6706, -8.9715)
  line L334 (-74.7956, -18.05) -> (-74.7956, -12.5)
  line L335 (-75.899, -10.9) -> (-73.5456, -10.9)
  line L336 (-43.6956, -10.9) -> (-41.3421, -10.9)
  line L337 (-41.3421, -9.7) -> (-43.6956, -9.7)
  arc A95 (-27.7171, -10.9) -> (-27.7171, -9.7) centre (-26.6206, -10.3) ccw
  line L338 (-69.6956, -12.5) -> (-69.6956, -18.05)
  line L339 (-47.5456, -18.05) -> (-47.5456, -12.5)
  line L340 (-59.9206, -27.6) -> (-59.9206, -28.3285)
  line L341 (-15.1956, -77.5) -> (-16.4456, -77.5)
  line L342 (-19.0456, -77.5) -> (-20.2956, -77.5)
  line L343 (-21.399, -79.1) -> (-19.0456, -79.1)
  line L344 (-16.4456, -79.1) -> (-14.0921, -79.1)
  line L345 (-14.0921, -80.3) -> (-16.4456, -80.3)
  line L346 (-19.0456, -80.3) -> (-21.399, -80.3)
  arc A96 (-19.0456, -81.0285) -> (-16.4456, -81.0285) centre (-17.7456, -82.2) ccw
  arc A97 (-14.0921, -80.3) -> (-14.0921, -79.1) centre (-12.9956, -79.7) ccw
  line L347 (-19.0456, -77.5) -> (-19.0456, -79.1)
  line L348 (-19.0456, -80.3) -> (-19.0456, -81.0285)
  line L349 (-16.4456, -81.0285) -> (-16.4456, -80.3)
  line L350 (-16.4456, -79.1) -> (-16.4456, -77.5)
  arc A98 (-21.399, -79.1) -> (-21.399, -80.3) centre (-22.4956, -79.7) ccw
  line L351 (-20.2956, -77.5) -> (-20.2956, -71.95)
  line L352 (-20.2956, -70.75) -> (-20.2956, -65.2)
  arc A99 (-21.399, -70.75) -> (-21.399, -71.95) centre (-22.4956, -71.35) ccw
  line L353 (-21.399, -70.75) -> (-20.2956, -70.75)
  line L354 (-15.1956, -70.75) -> (-14.0921, -70.75)
  line L355 (-14.0921, -71.95) -> (-15.1956, -71.95)
  line L356 (-20.2956, -71.95) -> (-21.399, -71.95)
  arc A100 (-14.0921, -71.95) -> (-14.0921, -70.75) centre (-12.9956, -71.35) ccw
  line L357 (-21.399, -63.6) -> (-19.0456, -63.6)
  line L358 (-16.4456, -63.6) -> (-14.0921, -63.6)
  line L359 (-14.0921, -62.4) -> (-16.4456, -62.4)
  line L360 (-19.0456, -62.4) -> (-21.399, -62.4)
  arc A101 (-16.4456, -61.6715) -> (-19.0456, -61.6715) centre (-17.7456, -60.5) ccw
  arc A102 (-14.0921, -63.6) -> (-14.0921, -62.4) centre (-12.9956, -63) ccw
  line L361 (-19.0456, -65.2) -> (-19.0456, -63.6)
  line L362 (-19.0456, -62.4) -> (-19.0456, -61.6715)
  arc A103 (-21.399, -62.4) -> (-21.399, -63.6) centre (-22.4956, -63) ccw
  line L363 (-20.2956, -65.2) -> (-19.0456, -65.2)
  line L364 (-16.4456, -65.2) -> (-15.1956, -65.2)
  line L365 (-16.4456, -61.6715) -> (-16.4456, -62.4)
  line L366 (-16.4456, -63.6) -> (-16.4456, -65.2)
  line L367 (-15.1956, -65.2) -> (-15.1956, -70.75)
  line L368 (-15.1956, -71.95) -> (-15.1956, -77.5)
  arc A104 (-19.0456, -54.6785) -> (-16.4456, -54.6785) centre (-17.7456, -55.85) ccw
  line L369 (-14.0921, -53.95) -> (-16.4456, -53.95)
  line L370 (-19.0456, -53.95) -> (-21.399, -53.95)
  line L371 (-16.4456, -54.6785) -> (-16.4456, -53.95)
  line L372 (-16.4456, -52.75) -> (-16.4456, -51.15)
  line L373 (-21.399, -52.75) -> (-19.0456, -52.75)
  line L374 (-16.4456, -52.75) -> (-14.0921, -52.75)
  line L375 (-19.0456, -51.15) -> (-19.0456, -52.75)
  line L376 (-19.0456, -53.95) -> (-19.0456, -54.6785)
  arc A105 (-21.399, -52.75) -> (-21.399, -53.95) centre (-22.4956, -53.35) ccw
  arc A106 (-14.0921, -53.95) -> (-14.0921, -52.75) centre (-12.9956, -53.35) ccw
  line L377 (-15.1956, -51.15) -> (-16.4456, -51.15)
  line L378 (-19.0456, -51.15) -> (-20.2956, -51.15)
  line L379 (-14.0921, -45.6) -> (-15.1956, -45.6)
  line L380 (-20.2956, -45.6) -> (-21.399, -45.6)
  line L381 (-21.399, -44.4) -> (-20.2956, -44.4)
  line L382 (-15.1956, -44.4) -> (-14.0921, -44.4)
  line L383 (-15.1956, -38.85) -> (-15.1956, -44.4)
  line L384 (-15.1956, -45.6) -> (-15.1956, -51.15)
  arc A107 (-14.0921, -45.6) -> (-14.0921, -44.4) centre (-12.9956, -45) ccw
  line L385 (-20.2956, -51.15) -> (-20.2956, -45.6)
  line L386 (-20.2956, -44.4) -> (-20.2956, -38.85)
  arc A108 (-21.399, -44.4) -> (-21.399, -45.6) centre (-22.4956, -45) ccw
  line L387 (-21.399, -37.25) -> (-19.0456, -37.25)
  line L388 (-16.4456, -37.25) -> (-14.0921, -37.25)
  line L389 (-20.2956, -38.85) -> (-19.0456, -38.85)
  line L390 (-16.4456, -38.85) -> (-15.1956, -38.85)
  line L391 (-19.0456, -38.85) -> (-19.0456, -37.25)
  line L392 (-19.0456, -36.05) -> (-19.0456, -35.3215)
  arc A109 (-21.399, -36.05) -> (-21.399, -37.25) centre (-22.4956, -36.65) ccw
  arc A110 (-16.4456, -35.3215) -> (-19.0456, -35.3215) centre (-17.7456, -34.15) ccw
  line L393 (-14.0921, -36.05) -> (-16.4456, -36.05)
  line L394 (-19.0456, -36.05) -> (-21.399, -36.05)
  arc A111 (-14.0921, -37.25) -> (-14.0921, -36.05) centre (-12.9956, -36.65) ccw
  line L395 (-16.4456, -35.3215) -> (-16.4456, -36.05)
  line L396 (-16.4456, -37.25) -> (-16.4456, -38.85)
  arc A112 (-19.0456, -28.3285) -> (-16.4456, -28.3285) centre (-17.7456, -29.5) ccw
  line L397 (-14.0921, -27.6) -> (-16.4456, -27.6)
  line L398 (-19.0456, -27.6) -> (-21.399, -27.6)
  line L399 (-21.399, -26.4) -> (-19.0456, -26.4)
  line L400 (-16.4456, -26.4) -> (-14.0921, -26.4)
  line L401 (-16.4456, -28.3285) -> (-16.4456, -27.6)
  line L402 (-16.4456, -26.4) -> (-16.4456, -24.8)
  arc A113 (-14.0921, -27.6) -> (-14.0921, -26.4) centre (-12.9956, -27) ccw
  line L403 (-19.0456, -24.8) -> (-19.0456, -26.4)
  line L404 (-19.0456, -27.6) -> (-19.0456, -28.3285)
  arc A114 (-21.399, -26.4) -> (-21.399, -27.6) centre (-22.4956, -27) ccw
  arc A115 (-14.0921, -19.25) -> (-14.0921, -18.05) centre (-12.9956, -18.65) ccw
  line L405 (-15.1956, -12.5) -> (-15.1956, -18.05)
  line L406 (-15.1956, -19.25) -> (-15.1956, -24.8)
  line L407 (-14.0921, -19.25) -> (-15.1956, -19.25)
  line L408 (-20.2956, -19.25) -> (-21.399, -19.25)
  line L409 (-21.399, -18.05) -> (-20.2956, -18.05)
  line L410 (-15.1956, -18.05) -> (-14.0921, -18.05)
  line L411 (-15.1956, -24.8) -> (-16.4456, -24.8)
  line L412 (-19.0456, -24.8) -> (-20.2956, -24.8)
  line L413 (-20.2956, -24.8) -> (-20.2956, -19.25)
  line L414 (-20.2956, -18.05) -> (-20.2956, -12.5)
  arc A116 (-21.399, -18.05) -> (-21.399, -19.25) centre (-22.4956, -18.65) ccw
  arc A117 (-16.4456, -8.9715) -> (-19.0456, -8.9715) centre (-17.7456, -7.8) ccw
  line L415 (-14.0921, -9.7) -> (-16.4456, -9.7)
  line L416 (-19.0456, -9.7) -> (-21.399, -9.7)
  line L417 (-21.399, -10.9) -> (-19.0456, -10.9)
  line L418 (-16.4456, -10.9) -> (-14.0921, -10.9)
  line L419 (-20.2956, -12.5) -> (-19.0456, -12.5)
  line L420 (-16.4456, -12.5) -> (-15.1956, -12.5)
  line L421 (-16.4456, -8.9715) -> (-16.4456, -9.7)
  line L422 (-16.4456, -10.9) -> (-16.4456, -12.5)
  arc A118 (-14.0921, -10.9) -> (-14.0921, -9.7) centre (-12.9956, -10.3) ccw
  line L423 (-19.0456, -12.5) -> (-19.0456, -10.9)
  line L424 (-19.0456, -9.7) -> (-19.0456, -8.9715)
  arc A119 (-21.399, -9.7) -> (-21.399, -10.9) centre (-22.4956, -10.3) ccw
  dimension "d74" = 12.3
  dimension "d82" = 5.55
  dimension "d88" = 2.5
  dimension "d89" = 2.5
  dimension "d93" = 1.25
  dimension "d95" = 5.1
  dimension "d98" = 2.2
  dimension "d103" = 1.6
  dimension "d104" = 2.5
  dimension "d105" = 2.5
  dimension "d106" = 3.5
  dimension "d107" = 4.7
  dimension "d113" = 45
  constraint vertical L351
  constraint horizontal L363
  constraint vertical L367
  constraint horizontal L355
  constraint horizontal L353
  constraint vertical L347
  constraint vertical L349
  constraint horizontal L345
  constraint horizontal L343
  constraint vertical L3
  constraint perpendicular L3 L4
  constraint collinear L5 L6
  constraint coincident L7.end L23
  constraint collinear L7 L8
  constraint coincident L9.end L11
  constraint collinear L9 L10
  constraint collinear L11 L12
  constraint collinear L13 L14
  constraint coincident L16.start L21
  constraint collinear L15 L16
  constraint coincident L18.start L19
  constraint collinear L17 L18
  constraint collinear L19 L20
  constraint collinear L21 L22
  constraint collinear L23 L24
  constraint coincident L26.start L29
  constraint collinear L25 L26
  constraint coincident L28.start L31
  constraint collinear L27 L28
  constraint collinear L29 L30
  constraint collinear L31 L32
  constraint coincident L33.start L39
  constraint coincident L36.start L35
  constraint collinear L35 L36
  constraint collinear L37 L38
  constraint collinear L39 L40
  constraint coincident L41.end L43
  constraint collinear L41 L42
  constraint coincident L43.end L113
  constraint collinear L43 L44
  constraint collinear L45 L46
  constraint collinear L47 L48
  constraint coincident L50.start L55
  constraint collinear L49 L50
  constraint coincident L52.start L53
  constraint collinear L51 L52
  constraint collinear L53 L54
  constraint collinear L55 L56
  constraint coincident L58.start L59
  constraint collinear L57 L58
  constraint collinear L59 L60
  constraint coincident L62.start L111
  constraint collinear L61 L62
  constraint collinear L63 L64
  constraint coincident L65.end L67
  constraint collinear L65 L66
  constraint coincident L67.end L71
  constraint collinear L67 L68
  constraint collinear L69 L70
  constraint collinear L71 L72
  constraint collinear L73 L74
  constraint coincident L76.start L81
  constraint collinear L75 L76
  constraint coincident L78.start L79
  constraint collinear L77 L78
  constraint collinear L79 L80
  constraint collinear L81 L82
  constraint coincident L84.start L89
  constraint collinear L83 L84
  constraint coincident L86.start L109
  constraint collinear L85 L86
  constraint collinear L87 L88
  constraint collinear L89 L90